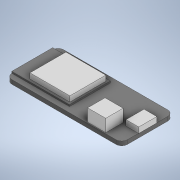
# Autodesk Inventor part: ESP32 Feather
Saved by Autodesk Inventor 2020 (Build 240168000, 168)
## iProperties
Created: 2019-11-26
Part Number: ESP32 Feather
Material: Generic
Document SubType Name: Modeling
Designer: Andrew
Density: 1 g/cm^3
Appearance: Default
PCB_Width: 22.950 mm
Author: Andrew
Autodesk Inventor part; units mm, degrees
ref_plane "YZ Plane" through (0, 0, 0) normal (1, 0, 0) x (0, 1, 0)
ref_plane "XZ Plane" through (0, 0, 0) normal (0, 1, 0) x (-1, 0, 0)
ref_plane "XY Plane" through (0, 0, 0) normal (0, 0, 1) x (1, 0, 0)
sketch "ESP32 Feather" plane through (0, 0, 0) normal (0, 0, 1) x (1, 0, 0)
  line L0 (-25.5, 0) -> (25.5, 0)
  line L1 (25.5, 0) -> (25.5, -1.8)
  line L2 (25.5, -1.8) -> (-25.5, -1.8)
  line L3 (-25.5, -1.8) -> (-25.5, 0)
  line L4 (0, 0) -> (-25.5, 0)
  line L5 (-25.5, 0) -> (-25.5, 0.75)
  line L6 (-25.5, 0.75) -> (0, 0.75)
  line L7 (0, 0.75) -> (0, 0)
  line L8 (-0.9, 0.75) -> (-18.55, 0.75)
  line L9 (-18.55, 0.75) -> (-18.55, 3.1)
  line L10 (-18.55, 3.1) -> (-0.9, 3.1)
  line L11 (-0.9, 3.1) -> (-0.9, 0.75)
  line L12 (10, 0) -> (18, 0)
  line L13 (18, 0) -> (18, 5.5)
  line L14 (18, 5.5) -> (10, 5.5)
  line L15 (10, 5.5) -> (10, 0)
  line L16 (25.6, 0) -> (19.95, 0)
  line L17 (19.95, 0) -> (19.95, 2.45)
  line L18 (19.95, 2.45) -> (25.6, 2.45)
  line L19 (25.6, 2.45) -> (25.6, 0)
  point P0 (0, 0)
  point P1 (0, 0)
  point P2 (-18.55, 0.75)
  point P3 (18, 0)
  point P4 (19.95, 0)
  dimension "d0" = 51
  dimension "d1" = 1.8
  dimension "d2" = 0.75
  dimension "d3" = 25.5
  dimension "d4" = 17.65
  dimension "d5" = 2.35
  dimension "d6" = 24.6
  dimension "d7" = 8
  dimension "d8" = 5.5
  dimension "d9" = 15.5
  dimension "d10" = 2.45
  dimension "d11" = 5.65
  dimension "d25" = 0.1
  constraints: 40 end point, 10 parallel, 5 horizontal, 5 perpendicular, 3 point on line, 2 midpoint, 1 coincident, 1 collinear
  measures "d0" distance of L1.end L2.end
  measures "d1" distance of L0.end L1.end
  measures "d2" distance of L6.end L4.start
  measures "d3" distance of L5.end L6.end
  measures "d4" distance of L9.end L10.end
  measures "d5" distance of L10.end L8.start
  measures "d6" distance between parallel lines of L5 L11
  measures "d7" distance of L13.end L14.end
  measures "d8" distance of L12.end L13.end
  measures "d9" distance between parallel lines of L1 L15
  measures "d10" distance of L16.start L18.end
  measures "d11" distance of L17.end L18.end
  measures "d25" distance between parallel lines of L1 L19
extrude "PCB" add sketch "ESP32 Feather" along normal mid plane 22.85 contours L0 L1 L2 L3
fillet "Fillet1" radius 2.5 4 edges at (-25.5, -0.9, 11.425) (-25.5, -0.9, -11.425) (25.5, -0.9, -11.425) (25.5, -0.9, 11.425)
extrude "ESP32PCB" add sketch "ESP32 Feather" along normal mid plane 18.1 contours L5 L6 L7 L0
extrude "ESP32Shied" add sketch "ESP32 Feather" along normal mid plane 15.9 contours L9 L10 L11 L6
extrude "Battery Connector" add sketch "ESP32 Feather" along normal blind 11 contours L15 L14 L13 L0
extrude "Extrusion5" cut sketch "ESP32 Feather" along normal blind 3.3 contours L15 L14 L13 L0
extrude "Extrusion6" add sketch "ESP32 Feather" along normal mid plane 8 contours L0 L17 L18 L19 L16
equation "\"d28\" = d26"
equation "\"d29\" = d26"
equation "\"PCB_Width\" = 22.95"
equation "\"d26\" = 1"
body "Solid1"
